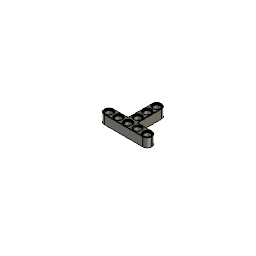
T-Element 5x5 (Autodesk Fusion 360 design; units mm, degrees)
Autodesk Fusion 360 part; units mm, degrees
sketch "Skizze1" plane through (0, 0, 0) normal (0, 0, 1) x (1, 0, 0)
  line L0 (19.9298, 0.1648) -> (19.9298, -0.0352)
  line L1 (16.1298, -3.8352) -> (-16.0702, -3.8352)
  line L2 (-19.8702, -0.0352) -> (-19.8702, 0.1648)
  circle A0 centre (-15.9702, 0.0648) radius 2.5
  circle A1 centre (-15.9702, 0.0648) radius 3.2
  line L3 (3.9298, -3.8352) -> (-3.8702, -3.8352)
  line L4 (-0.0702, 27.9648) -> (0.1298, 27.9648)
  circle A2 centre (-7.9702, 0.0648) radius 2.5
  circle A3 centre (-7.9702, 0.0648) radius 3.2
  circle A4 centre (0.0298, 0.0648) radius 2.5
  circle A5 centre (0.0298, 0.0648) radius 3.2
  circle A6 centre (8.0298, 0.0648) radius 2.5
  circle A7 centre (8.0298, 0.0648) radius 3.2
  circle A8 centre (16.0298, 0.0648) radius 2.5
  circle A9 centre (16.0298, 0.0648) radius 3.2
  circle A10 centre (0.0298, 8.0648) radius 2.5
  circle A11 centre (0.0298, 8.0648) radius 3.2
  circle A12 centre (0.0298, 16.0648) radius 2.5
  circle A13 centre (0.0298, 16.0648) radius 3.2
  circle A14 centre (0.0298, 24.0648) radius 2.5
  circle A15 centre (0.0298, 24.0648) radius 3.2
  arc A16 (-0.0702, 27.9648) -> (-3.8702, 24.1648) centre (-0.0702, 24.1648) ccw
  arc A17 (3.9298, 24.1648) -> (0.1298, 27.9648) centre (0.1298, 24.1648) ccw
  arc A18 (19.9298, 0.1648) -> (16.1298, 3.9648) centre (16.1298, 0.1648) ccw
  arc A19 (16.1298, -3.8352) -> (19.9298, -0.0352) centre (16.1298, -0.0352) ccw
  arc A20 (-19.8702, -0.0352) -> (-16.0702, -3.8352) centre (-16.0702, -0.0352) ccw
  arc A21 (-16.0702, 3.9648) -> (-19.8702, 0.1648) centre (-16.0702, 0.1648) ccw
  line L5 (-3.8702, 4.9648) -> (-3.8702, 24.1648)
  line L6 (3.9298, 24.1648) -> (3.9298, 4.9648)
  line L7 (19.9298, 0.0648) -> (18.5298, 0.0648)
  line L8 (5.5298, 0.0648) -> (4.8298, 0.0648)
  line L9 (-16.0702, 3.9648) -> (-4.8702, 3.9648)
  line L10 (4.9298, 3.9648) -> (16.1298, 3.9648)
  arc A22 (-4.8702, 3.9648) -> (-3.8702, 4.9648) centre (-4.8702, 4.9648) ccw
  arc A23 (3.9298, 4.9648) -> (4.9298, 3.9648) centre (4.9298, 4.9648) ccw
  point P0 (-19.8702, 3.9648)
  point P1 (19.9298, 3.9648)
  point P2 (-19.8702, -3.8352)
  point P3 (3.9298, 27.9648)
  dimension "d1" = 7.8
  dimension "d2" = 39.8
  dimension "d3" = 5
  dimension "d4" = 6.4
  dimension "d5" = 7.8
  dimension "d6" = 31.8
  dimension "d7" = 3.9
  dimension "d8" = 3.9
  dimension "d10" = 16
  dimension "d13" = 32
  dimension "d14" = 0
  dimension "d17" = 0
  dimension "d18" = 24
  dimension "d19" = 3.8
  dimension "d20" = 1
  constraint horizontal L9
  constraint vertical L0
  constraint horizontal L1
  constraint vertical L2
  constraint concentric A0 A1
  constraint horizontal L3
  constraint horizontal L4
  constraint vertical L6
  constraint coincident L1 L3.start
  constraint tangent L4 A16
  constraint coincident P3 L4
  constraint coincident P3 L6
  constraint tangent L4 A17
  constraint tangent A17 L6
  constraint equal A16 A17
  constraint coincident L0 L7.start
  constraint coincident P1 L9
  constraint coincident P1 L0
  constraint tangent A18 L9
  constraint tangent L0 A18
  constraint equal A16 A18
  constraint tangent L0 A19
  constraint tangent L1 A19
  constraint equal A16 A19
  constraint coincident P2 L1
  constraint coincident P2 L2
  constraint tangent L1 A20
  constraint tangent L2 A20
  constraint equal A16 A20
  constraint coincident P0 L9
  constraint coincident P0 L2
  constraint tangent A21 L9
  constraint tangent L2 A21
  constraint equal A16 A21
  constraint coincident A7 L8.end
  constraint coincident A6 L8.start
  constraint collinear L7 L8
  constraint coincident A8 L7.end
  constraint collinear L9 L10
  constraint tangent L9 A22
  constraint tangent L5 A22
  constraint tangent L6 A23
  constraint tangent L10 A23
  constraint equal A22 A23
  measures "d1" distance of P0 P2
  measures "d2" distance of P0 P1
  measures "d3" diameter of A0
  measures "d4" diameter of A1
  measures "d5" distance of L3.start L3.end
  measures "d6" distance of L3.start P3
  measures "d7" distance of A0.centre L9
  measures "d8" distance of L2 A0.centre
  measures "d10" distance of L0 L6
  measures "d19" radius of A16
  measures "d20" radius of A22
extrude "Extrusion1" add sketch "Skizze1" along normal blind 7.8 contours L0 L1 L2 L3 L4 A16 A17 A18 A19 A20 A21 L5 L6 L9 L10 A22 A23
extrude "Extrusion2" add sketch "Skizze1" along normal blind 6.2 from surface at 0.8 contours A1 | A3 | A5 | A7 | A9 | A11 | A13 | A15
fillet "Abrundung1" radius 0.2 77 edges at (-10.4702, 3.9648, 7.8) (-18.7572, 2.8518, 7.8) (-19.8702, 0.0648, 7.8) (-18.7572, -2.7222, 7.8) (0.0298, -3.8352, 7.8) (18.8169, -2.7222, 7.8) (19.9298, 0.0648, 7.8) (18.8169, 2.8518, 7.8) (10.5298, 3.9648, 7.8) (4.2227, 4.2577, 7.8) (3.9298, 14.5648, 7.8) (2.8169, 26.8518, 7.8) (0.0298, 27.9648, 7.8) (-2.7572, 26.8518, 7.8) (-3.8702, 14.5648, 7.8) (-4.163, 4.2577, 7.8) (-2.7572, 26.8518, 0) (-3.8702, 14.5648, 0) (-4.163, 4.2577, 0) (-10.4702, 3.9648, 0) (-18.7572, 2.8518, 0) (-19.8702, 0.0648, 0) (-18.7572, -2.7222, 0) (0.0298, -3.8352, 0) (18.8169, -2.7222, 0) (19.9298, 0.0648, 0) (18.8169, 2.8518, 0) (10.5298, 3.9648, 0) (4.2227, 4.2577, 0) (3.9298, 14.5648, 0) (2.8169, 26.8518, 0) (0.0298, 27.9648, 0) (-2.9536, 1.222, 7.8) (-2.9536, 1.222, 7) (-2.301, 0.9689, 7) (-10.9536, 1.222, 7.8) (-10.301, 0.9689, 7) (-10.9536, 1.222, 7) (-18.9536, 1.222, 7.8) (-18.9536, 1.222, 7) (-18.301, 0.9689, 7) (-2.9536, 9.222, 7.8) (-2.9536, 9.222, 7) (-2.301, 8.9689, 7) (-2.9536, 17.222, 7.8) (-2.9536, 17.222, 7) (-2.301, 16.9689, 7) (-2.9536, 25.222, 7.8) (-2.9536, 25.222, 7) (-2.301, 24.9689, 7) (13.0464, 1.222, 7.8) (13.699, 0.9689, 7) (13.0464, 1.222, 7) (13.0464, 1.222, 0) (13.699, 0.9689, 0.8) (13.0464, -1.0924, 0.8) (5.699, 0.9689, 0.8) (5.0464, -1.0924, 0.8) (5.0464, 1.222, 0) (-2.9536, 1.222, 0) (-2.9536, -1.0924, 0.8) (-2.301, 0.9689, 0.8) (-10.9536, 1.222, 0) (-10.9536, -1.0924, 0.8) (-10.301, 0.9689, 0.8) (-18.9536, 1.222, 0) (-18.9536, -1.0924, 0.8) (-18.301, 0.9689, 0.8) (-2.9536, 9.222, 0) (-2.301, 8.9689, 0.8) (-2.9536, 6.9076, 0.8) (-2.9536, 17.222, 0) (-2.9536, 14.9076, 0.8) (-2.301, 16.9689, 0.8) (-2.9536, 25.222, 0) (-2.301, 24.9689, 0.8) (-2.9536, 22.9076, 0.8)
named bodies: "T-Element 5x5"
